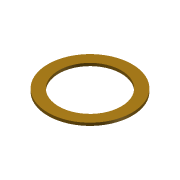
# Autodesk Inventor part: real
Saved by Autodesk Inventor 2012 SP2 (Build 160219200, 219)
## iProperties
Created: 2011-12-05
Material: 黃銅，淡黃
Document SubType Name: Modeling
Designer: Eric
Density: 8.47 g/cm^3
Mass: 0.33487 g
Surface Area: 1.9922 cm^2
Volume: 0.039536 cm^3
Description: 黃銅墊片
Author: Eric
Autodesk Inventor part; units mm, degrees
ref_plane "YZ Plane" through (0, 0, 0) normal (1, 0, 0) x (0, 1, 0)
ref_plane "XZ Plane" through (0, 0, 0) normal (0, 1, 0) x (-1, 0, 0)
ref_plane "XY Plane" through (0, 0, 0) normal (0, 0, 1) x (1, 0, 0)
sketch "草圖1" plane through (0, 0, 0) normal (0, 0, 1) x (1, 0, 0)
  circle A0 centre (0, 0) radius 5.575
  circle A1 centre (0, 0) radius 7.5
  dimension "d0" = 11.15
  dimension "d1" = 15
  constraints: 2 centre point, 2 coincident
  measures "d0" diameter of A0
  measures "d1" diameter of A1
extrude "擠出1" add sketch "草圖1" along normal blind 0.5
